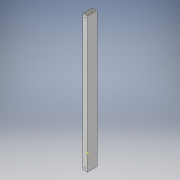
# Autodesk Inventor part: 2x1 20in Alluminum.ver1-1111-2019
Saved by Autodesk Inventor 2018 (Build 220112000, 112)
## iProperties
Created: 2019-10-10
Part Number: 2x1 20in Alluminum.ver1-1111-2019
Material: Generic
Document SubType Name: Modeling
Designer: JMHal
Density: 1 g/cm^3
Appearance: Default
Author: JMHal
Autodesk Inventor part; units mm, degrees
ref_plane "YZ Plane" through (0, 0, 0) normal (1, 0, 0) x (0, 1, 0)
ref_plane "XZ Plane" through (0, 0, 0) normal (0, 1, 0) x (-1, 0, 0)
ref_plane "XY Plane" through (0, 0, 0) normal (0, 0, 1) x (1, 0, 0)
sketch "Sketch1" plane through (0, 0, 0) normal (0, 1, 0) x (-1, 0, 0)
  line L0 (0, 0) -> (25.4, 0)
  line L1 (25.4, 0) -> (25.4, -50.8)
  line L2 (25.4, -50.8) -> (0, -50.8)
  line L3 (0, -50.8) -> (0, 0)
  line L4 (22.225, -47.625) -> (22.225, -3.175)
  line L5 (22.225, -3.175) -> (3.175, -3.175)
  line L6 (3.175, -3.175) -> (3.175, -47.625)
  line L7 (3.175, -47.625) -> (22.225, -47.625)
  dimension "d0" = 25.4
  dimension "d1" = 50.8
  dimension "d2" = 3.175
  constraints: 16 end point, 4 parallel, 2 perpendicular, 1 horizontal, 3 other
  measures "d0" distance of L1.end L2.end
  measures "d1" distance of L0.end L1.end
  measures "d2" distance between parallel lines of L1 L4
extrude "Extrusion1" add sketch "Sketch1" along normal blind 533.4
sketch "Sketch2" plane through (0, 0, 0) normal (1, 0, 0) x (0, 0, -1)
  point P0 (0, 0)
sketch "Sketch3" plane through (0, 0, 0) normal (0, -1, 0) x (1, 0, 0)
  line L0 (-3.175, -47.625) -> (-22.225, -47.625) projected
  line L1 (-22.225, -47.625) -> (-22.225, -3.175) projected
  line L2 (-22.225, -3.175) -> (-3.175, -3.175) projected
  line L3 (-3.175, -3.175) -> (-3.175, -47.625) projected
  line L4 (0, 0) -> (-25.4, 0) projected
  line L5 (-25.4, 0) -> (-25.4, -50.8) projected
  line L6 (-25.4, -50.8) -> (0, -50.8) projected
  line L7 (0, -50.8) -> (0, 0) projected
extrude "Extrusion2" add sketch "Sketch3" along normal blind 88.9
sketch "Sketch4" plane through (0, 533.4, 0) normal (0, 1, 0) x (1, 0, 0)
  line L0 (-22.225, 47.625) -> (-3.175, 47.625) projected
  line L1 (-3.175, 47.625) -> (-3.175, 3.175) projected
  line L2 (-3.175, 3.175) -> (-22.225, 3.175) projected
  line L3 (-22.225, 3.175) -> (-22.225, 47.625) projected
  line L4 (-25.4, 0) -> (0, 0) projected
  line L5 (0, 0) -> (0, 50.8) projected
  line L6 (0, 50.8) -> (-25.4, 50.8) projected
  line L7 (-25.4, 50.8) -> (-25.4, 0) projected
extrude "Extrusion3" add sketch "Sketch4" along normal blind 88.9
sketch "Sketch6" plane through (0, -88.9, 0) normal (1, 0, 0) x (0, 0, -1)
  line L0 (29.7808, 711.2) -> (29.7808, 547.6875) projected
  line L1 (50.8, 711.2) -> (50.8, 0) projected
  line L2 (0, 711.2) -> (50.8, 711.2) projected
  line L3 (0, 0) -> (0, 711.2) projected
  line L4 (50.8, 0) -> (0, 0) projected
  line L5 (0, 0) -> (0, 711.2) projected
  line L6 (0, 711.2) -> (50.8, 711.2)
  line L7 (50.8, 711.2) -> (50.8, 685.8)
  line L8 (50.8, 685.8) -> (0, 685.8)
  line L9 (0, 685.8) -> (0, 711.2)
  point P0 (0, 88.9)
  dimension "d14" = 25.4
  constraints: 8 end point, 2 parallel, 1 horizontal, 1 perpendicular, 1 point on line
  measures "d14" distance between parallel lines of L2 L8
extrude "Extrusion5" cut sketch "Sketch6" against normal blind 25.4 contours L2 L1 L8 L0 | L0 L8 L3 L2
sketch "Sketch7" plane through (0, 596.9, 0) normal (0, 1, 0) x (1, 0, 0)
  line L0 (-3.175, 47.625) -> (-22.225, 47.625) projected
  line L1 (-3.175, 3.175) -> (-3.175, 47.625) projected
  line L2 (-22.225, 3.175) -> (-3.175, 3.175) projected
  line L3 (-22.225, 47.625) -> (-22.225, 3.175) projected
  line L4 (0, 50.8) -> (0, 0) projected
  line L5 (-25.4, 50.8) -> (0, 50.8) projected
  line L6 (-25.4, 0) -> (-25.4, 50.8) projected
  line L7 (0, 0) -> (-25.4, 0) projected
  point P0 (0, 0)
extrude "Extrusion6" add sketch "Sketch7" along normal blind 25.4
sketch "Sketch8" plane through (-25.4, -88.9, 0) normal (0, 0, 1) x (1, 0, 0)
  point P0 (25.4, 88.9)
sketch "Sketch9" plane through (-25.4, -88.9, 0) normal (0, 0, 1) x (1, 0, 0)
  circle A0 centre (12.7, 12.7) radius 2.0701
  line L0 (25.4, 0) -> (0, 0) projected
  line L1 (25.4, 0) -> (25.4, 711.2) projected
  point P0 (25.4, 88.9)
  dimension "d19" = 4.1402
  dimension "d20" = 12.7
  dimension "d21" = 12.7
  constraints: 1 centre point
  measures "d19" diameter of A0
  measures "d20" distance from line of A0.centre L0
  measures "d21" distance from line of A0.centre L1
extrude "Extrusion7" cut sketch "Sketch9" against normal blind 25.4
sketch "Sketch10" plane through (-25.4, -88.9, 0) normal (0, 0, 1) x (1, 0, 0)
  circle A0 centre (12.7, 698.5) radius 2.0701
  line L0 (0, 711.2) -> (25.4, 711.2) projected
  line L1 (0, 711.2) -> (0, 0) projected
  point P0 (25.4, 88.9)
  dimension "d24" = 4.1402
  dimension "d25" = 12.7
  dimension "d26" = 12.7
  constraints: 1 centre point
  measures "d24" diameter of A0
  measures "d25" distance from line of A0.centre L0
  measures "d26" distance from line of A0.centre L1
extrude "Extrusion8" cut sketch "Sketch10" against normal blind 25.4
body "Solid1"
